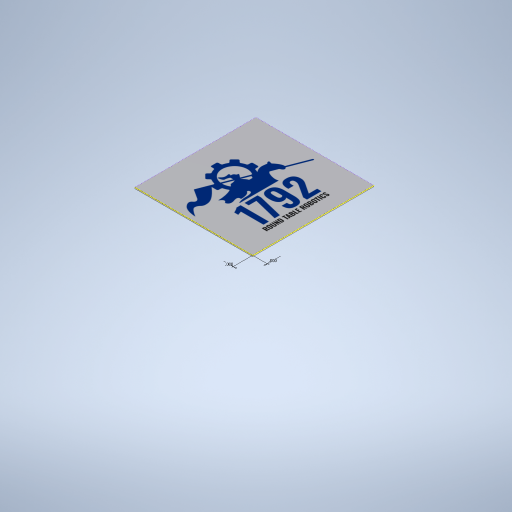
# Autodesk Inventor part: 1792
Saved by Autodesk Inventor 2023 (Build 270158000, 158)
## iProperties
Created: 2023-12-23
Part Number: 1792
Material: Generic
Document SubType Name: Sheet Metal
Designer: elija
Density: 1 g/cm^3
Sheet Metal Rule: Default
Appearance: Default
Author: elija
Autodesk Inventor part; units mm, degrees
ref_plane "YZ Plane" through (0, 0, 0) normal (1, 0, 0) x (0, 1, 0)
ref_plane "XZ Plane" through (0, 0, 0) normal (0, 1, 0) x (-1, 0, 0)
ref_plane "XY Plane" through (0, 0, 0) normal (0, 0, 1) x (1, 0, 0)
sketch "Sketch1" plane through (0, 0, 0) normal (0, 1, 0) x (-1, 0, 0)
  line L0 (0, 0) -> (304.8, 0)
  line L1 (304.8, 0) -> (304.8, -313.4412)
  line L2 (304.8, -313.4412) -> (0, -313.4412)
  line L3 (0, -313.4412) -> (0, 0)
  point P0 (0, 0)
  dimension "d59" = 304.8
  dimension "d60" = 313.4412
  measures "d59" distance of L0.start L0.end
  measures "d60" distance of L2.end L0.start
extrude "Plate1" add sketch "Sketch1" against normal blind 3.048
sketch "Sketch2" plane through (0, 0, 0) normal (0, 1, 0) x (1, 0, 0)
  line L0 (-304.8, 0) -> (-304.8, 313.4412) construction
  line L1 (-304.8, 313.4412) -> (0, 313.4412) construction
  line L2 (0, 313.4412) -> (0, 0) construction
  line L3 (0, 0) -> (-304.8, 0) construction
  line L4 (0, 0) -> (0, 313.4412) projected
  line L5 (-304.8, 0) -> (0, 0) projected
  dimension "d63" = 0
  dimension "d64" = 0
  constraints: 2 other
  measures "d63" distance between parallel lines of L4 L2
  measures "d64" distance between parallel lines of L5 L3
equation "\"d58\" = Thickness"
equation "\"BendRadius\" = Thickness"
equation "\"BendReliefWidth\" = Thickness"
equation "\"BendReliefDepth\" = 0.5 * Thickness"
equation "\"CornerReliefSize\" = 4 * Thickness"
equation "\"MinimumRemnant\" = 2 * Thickness"
equation "\"TransitionRadius\" = BendRadius"
equation "\"JacobiRadiusSize\" = BendRadius"
equation "\"GapSize\" = Thickness"
equation "\"Thickness\" = 3.048"
body "Solid1"
